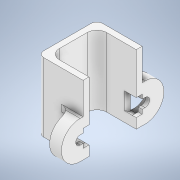
# Autodesk Inventor part: Pololu_MicroMotorMount
Saved by Autodesk Inventor 2021 (Build 250183000, 183)
## iProperties
Created: 2022-05-16
Part Number: Pololu_MicroMotorMount
Material: Generic
Document SubType Name: Modeling
Designer: ermoz
Density: 1 g/cm^3
Appearance: Default
Author: ermoz
Autodesk Inventor part; units mm, degrees
ref_plane "YZ Plane" through (0, 0, 0) normal (1, 0, 0) x (0, 1, 0)
ref_plane "XZ Plane" through (0, 0, 0) normal (0, 1, 0) x (-1, 0, 0)
ref_plane "XY Plane" through (0, 0, 0) normal (0, 0, 1) x (1, 0, 0)
sketch "Sketch1" plane through (0, 0, 0) normal (0, 1, 0) x (-1, 0, 0)
  line L0 (0, 0) -> (0, -1.5)
  line L1 (0, -1.5) -> (10, -1.5)
  line L2 (10, -1.5) -> (10, -13.5)
  line L3 (10, -13.5) -> (0, -13.5)
  line L4 (0, -13.5) -> (0, -15)
  line L5 (0, -15) -> (11.5, -15)
  line L6 (11.5, -15) -> (11.5, 0)
  line L7 (11.5, 0) -> (0, 0)
  dimension "d0" = 1.5
  dimension "d1" = 1.5
  dimension "d2" = 1.5
  dimension "d3" = 10
  dimension "d4" = 12
  constraints: 16 end point, 6 perpendicular, 2 point on line, 1 vertical
  measures "d0" distance between parallel lines of L7 L1
  measures "d1" distance between parallel lines of L6 L2
  measures "d2" distance between parallel lines of L5 L3
  measures "d3" distance of L0.end L1.end
  measures "d4" distance of L1.end L2.end
extrude "Extrusion1" add sketch "Sketch1" along normal blind 17.5
fillet "Fillet1" radius 1.5 2 edges at (-11.5, 8.75, 0) (-11.5, 8.75, -15)
fillet "Fillet2" radius 2.5 2 edges at (-10, 8.75, -13.5) (-10, 8.75, -1.5)
sketch "Sketch2" plane through (0, 0, 0) normal (0, -1, 0) x (1, 0, 0)
  line L0 (0, 0) -> (-3, 0)
  line L1 (-3, 0) -> (-3, 5.5)
  line L2 (-3, 5.5) -> (0, 5.5)
  line L3 (0, 5.5) -> (0, 0)
  line L4 (0, -15) -> (-10, -15) projected
  line L5 (0, -15) -> (-3, -15)
  line L6 (-3, -15) -> (-3, -20.5)
  line L7 (-3, -20.5) -> (0, -20.5)
  line L8 (0, -20.5) -> (0, -15)
  dimension "d9" = 3
  dimension "d10" = 5.5
  constraints: 16 end point, 4 parallel, 2 horizontal, 2 perpendicular, 1 collinear, 1 point on line
  measures "d9" distance of L1.end L2.end
  measures "d10" distance of L2.end L0.start
extrude "Extrusion2" add sketch "Sketch2" against normal blind 9.5
fillet "Fillet3" radius 4.75 4 edges at (-1.5, 0, 5.5) (-1.5, 9.5, 5.5) (-1.5, 0, -20.5) (-1.5, 9.5, -20.5)
fillet "Fillet4" radius 2.5 2 edges at (-3, 4.75, -15) (-3, 4.75, 0)
sketch "Sketch3" plane through (-3, 4.75, -15.75) normal (-1, 0, 0) x (0, 0, 1)
  arc A0 (0, 4.75) -> (0, -4.75) centre (0, 0) ccw projected
  circle A1 centre (0, 0) radius 3.5
  line L0 (-3.0311, -1.75) -> (-3.0311, 1.75)
  line L1 (-3.0311, 1.75) -> (0, 3.5)
  line L2 (0, 3.5) -> (3.0311, 1.75)
  line L3 (3.0311, 1.75) -> (3.0311, -1.75)
  line L4 (3.0311, -1.75) -> (0, -3.5)
  line L5 (0, -3.5) -> (-3.0311, -1.75)
  line L6 (2.25, -4.75) -> (2.25, 12.75) projected
  circle A2 centre (0, 0) radius 1.125
  line L7 (0.75, -4.75) -> (0.75, 4.75) projected
  line L8 (0.75, 3.067) -> (0.75, -3.067)
  arc A3 (18.25, -4.4159) -> (18.25, 4.4159) centre (16.5, 0) ccw projected
  line L9 (19.5311, 1.75) -> (19.5311, -1.75)
  line L10 (19.5311, -1.75) -> (16.5, -3.5)
  line L11 (16.5, -3.5) -> (13.4689, -1.75)
  line L12 (13.4689, -1.75) -> (13.4689, 1.75)
  line L13 (13.4689, 1.75) -> (16.5, 3.5)
  line L14 (16.5, 3.5) -> (19.5311, 1.75)
  line L15 (14.25, 12.75) -> (14.25, -4.75) projected
  line L16 (15.75, -4.75) -> (15.75, 12.75) projected
  line L17 (15.75, -3.067) -> (15.75, 3.067)
  circle A4 centre (16.5, 0) radius 1.125
  point P0 (2.25, -2.201)
  point P1 (2.25, 2.201)
  point P2 (0.75, 0.8385)
  point P3 (0.75, -0.8385)
  point P4 (15.75, 0.8385)
  point P5 (15.75, -0.8385)
  point P6 (14.25, 2.201)
  point P7 (14.25, -2.201)
  dimension "d15" = 3.5
  dimension "d16" = 2.25
  dimension "d25" = 2.25
  constraints: 28 end point, 8 point on line, 5 coincident, 3 parallel, 2 centre point, 29 other
  measures "d15" distance of L0.start L0.end
  measures "d16" diameter of A2
  measures "d25" diameter of A4
extrude "Extrusion3" cut sketch "Sketch3" along normal blind 10 and the other way blind 2 contours L7 A2 L4 L5 L0 L1 L2 | L7 A2 | L9 L10 L11 L16 A4 L13 L14 | A4 L16 picked at (0.2626, -0.3643) picked at (16.8752, 0.2073)
extrude "Extrusion4" cut sketch "Sketch3" against normal through all contours L7 A2 | A2 L7 | A4 L16 | L16 A4
extrude "Extrusion5" cut sketch "Sketch3" against normal up to surface (2 mm away) contours L6 L4 L7 A2 L2 | L16 A4 L11 L15 L13
sketch "Sketch4" plane through (0, 0, -13.5) normal (1, 0, 0) x (0, 0, -1)
  circle A0 centre (2.25, 4.75) radius 1.125 projected
  line L0 (2.25, 5.875) -> (-14.25, 5.875)
  line L1 (-14.25, 5.875) -> (-14.25, 3.625)
  line L2 (-14.25, 3.625) -> (2.25, 3.625)
  line L3 (2.25, 3.625) -> (2.25, 5.875)
  circle A1 centre (-14.25, 4.75) radius 1.125 projected
  point P0 (-13.5, 0)
  point P1 (2.25, 3.625)
  constraints: 8 end point, 2 parallel, 2 tangent, 1 horizontal, 1 midpoint, 1 perpendicular, 2 other
extrude "Extrusion6" cut sketch "Sketch4" against normal up to surface (1 mm away) contours A0 L2 A1 L0
sketch "Sketch5" plane through (0, 17.5, 0) normal (1, 0, 0) x (0, 0, -1)
  line L0 (0, -17.5) -> (0, 0) projected
  line L1 (15, -9.683) -> (15, -15.817) projected
  line L2 (0, -10.549) -> (15, -10.549)
  line L3 (15, -10.549) -> (15, -14.951)
  line L4 (15, -14.951) -> (0, -14.951)
  line L5 (0, -14.951) -> (0, -10.549)
  point P0 (13.5, -14.951)
  point P1 (1.5, -10.549)
  point P2 (0, -14.951)
  constraints: 8 end point, 4 point on line, 2 parallel, 1 horizontal, 1 perpendicular
extrude "Extrusion7" cut sketch "Sketch5" against normal up to surface (3 mm away)
body "Solid1"
